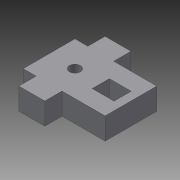
# Autodesk Inventor part: Frame_Upper_Vertical_Plate_A
Saved by Autodesk Inventor 2014 (Build 180170000, 170)
## iProperties
Created: 2014-08-27
Part Number: Frame_Upper_Vertical_Plate_A
Material: Generic
Document SubType Name: Modeling
Designer: ThatOtherGuy
Density: 1 g/cm^3
Appearance: Default
Author: ThatOtherGuy
Autodesk Inventor part; units mm, degrees
ref_plane "YZ Plane" through (0, 0, 0) normal (1, 0, 0) x (0, 1, 0)
ref_plane "XZ Plane" through (0, 0, 0) normal (0, 1, 0) x (-1, 0, 0)
ref_plane "XY Plane" through (0, 0, 0) normal (0, 0, 1) x (1, 0, 0)
sketch "Sketch1" plane through (0, 0, 0) normal (0, 0, 1) x (1, 0, 0)
  line L0 (0, 0) -> (3.75, 0)
  line L1 (3.75, 0) -> (3.75, -5)
  line L2 (3.75, -5) -> (11.25, -5)
  line L3 (11.25, -5) -> (11.25, 0)
  line L4 (11.25, 0) -> (23.75, 0)
  line L5 (23.75, 0) -> (23.75, 15)
  line L6 (23.75, 15) -> (11.25, 15)
  line L7 (11.25, 15) -> (11.25, 20)
  line L8 (11.25, 20) -> (3.75, 20)
  line L9 (3.75, 20) -> (3.75, 15)
  line L10 (3.75, 15) -> (0, 15)
  line L11 (0, 15) -> (0, 0)
  line L12 (21.731, 10) -> (15, 10)
  line L13 (15, 10) -> (15, 5)
  line L14 (15, 5) -> (21.731, 5)
  line L15 (21.731, 5) -> (21.731, 10)
  circle A0 centre (7.5, 7.5) radius 1.6
  point P0 (21.731, 7.5)
  point P1 (23.75, 7.5)
  point P2 (7.5, -5)
  point P3 (0, 7.5)
  dimension "d0" = 15
  dimension "d1" = 3.75
  dimension "d2" = 5
  dimension "d3" = 7.5
  dimension "d4" = 12.5
  dimension "d5" = 6.731
  dimension "d6" = 5
  dimension "d7" = 3.75
  dimension "d12" = 3.2
  constraints: 32 end point, 10 parallel, 5 equal length, 4 midpoint, 2 collinear, 2 horizontal, 2 horizontal alignment, 2 perpendicular, 1 centre point, 1 vertical alignment
  measures "d0" distance of L10.end L0.start
  measures "d1" distance of L0.start L0.end
  measures "d2" distance of L0.end L1.end
  measures "d3" distance of L7.end L8.end
  measures "d4" distance of L5.end L6.end
  measures "d5" distance of L12.start L12.end
  measures "d6" distance of L12.end L13.end
  measures "d7" distance between parallel lines of L3 L13
  measures "d12" diameter of A0
extrude "Extrusion1" add sketch "Sketch1" along normal blind 6.731
equation "\"d5\" = THICKB"
equation "\"d7\" = d1"
equation "\"d8\" = THICKB"
equation "\"THICKA\" = 3.175"
equation "\"THICKB\" = 6.731"
equation "\"THICKC\" = 12.7"
equation "\"MAGDIA\" = 9.5"
equation "\"BALLDIA\" = 12"
equation "\"THICKPLY\" = 5"
body "Solid1"
